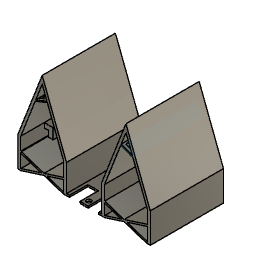
V shape load bearer v7 (Autodesk Fusion 360 design; units mm, degrees)
Autodesk Fusion 360 part; units mm, degrees
sketch "Sketch1" plane through (0, 0, 0) normal (0, 0, 1) x (1, 0, 0)
  line L0 (0, 0) -> (66, 0)
  line L1 (66, 0) -> (66, 150)
  line L2 (66, 150) -> (0, 150)
  line L3 (0, 150) -> (0, 0)
  dimension "d3" = 150
  dimension "d4" = 66
  constraint horizontal L0
  constraint vertical L1
  constraint horizontal L2
  constraint vertical L3
  constraint coincident L0.start L3.end
  measures "d3" distance of L0.start L2.end
  measures "d4" distance of L0.start L0.end
extrude "Extrude1" add sketch "Sketch1" along normal blind 2 makes body 1
sketch "Sketch2" plane through (0, 0, 2) normal (0, 0, 1) x (-1, 0, 0)
  line L0 (0, -150) -> (0, 0)
  line L1 (0, 0) -> (-66, 0)
  line L2 (-66, 0) -> (-66, -150)
  line L3 (-66, -150) -> (0, -150)
  line L4 (0, 0) -> (-3, 0)
  line L5 (-3, 0) -> (-3, -150)
  line L6 (-3, -150) -> (0, -150)
  line L7 (0, -150) -> (0, 0)
  line L8 (-66, -150) -> (-63, -150)
  line L9 (-63, -150) -> (-63, 0)
  line L10 (-63, 0) -> (-66, 0)
  line L11 (-66, 0) -> (-66, -150)
  dimension "d5" = 3
  dimension "d6" = 3
  constraint horizontal L4
  constraint vertical L5
  constraint horizontal L6
  constraint vertical L7
  constraint coincident L3 L5.end
  constraint coincident L0.end L1.start
  constraint horizontal L8
  constraint vertical L9
  constraint horizontal L10
  constraint vertical L11
  constraint coincident L1 L9.end
  constraint coincident L2.end L3.start
  measures "d5" distance of L0.end L4.end
  measures "d6" distance of L2.end L8.end
extrude "Extrude2" add sketch "Sketch2" along normal blind 40 contours L0 L1 L3 L4 L5 L6 L7 | L1 L2 L3 L8 L9 L10 L11 bodies 1
extrude "Extrude3" add 1 faces at (0, 100, 28) along direction (-1, 0, 0) blind 60 on bodies 1 bodies 1
extrude "Extrude4" add 1 faces at (66, 50, 28) along direction (1, 0, 0) blind 60 on bodies 1 bodies 1
sketch "Sketch3" plane through (0, 0, 0) normal (0, 0, -1) x (1, 0, 0)
  line L0 (-60, -150) -> (126, -150)
  line L1 (126, -150) -> (126, 0)
  line L2 (126, 0) -> (-60, 0)
  line L3 (-60, 0) -> (-60, -150)
  line L4 (-50, -10) -> (0, -10)
  line L5 (0, -10) -> (0, -140)
  line L6 (0, -140) -> (-50, -140)
  line L7 (-50, -140) -> (-50, -10)
  constraint horizontal L4
  constraint vertical L5
  constraint horizontal L6
  constraint vertical L7
extrude "Extrude5" cut sketch "Sketch3" against normal blind 38 contours L4 L5 L6 L7 bodies 1
extrude "Extrude6" cut 1 faces at (-50, 96.6667, 12.6667) along direction (-1, 0, 0) blind 5 on bodies 1 bodies 1
extrude "Extrude7" add 1 faces at (0, 53.3333, 12.6667) along direction (-1, 0, 0) blind 2 on bodies 1 bodies 1
extrude "Extrude8" add 1 faces at (-60, 100, 28) along direction (-1, 0, 0) blind 20 on bodies 1 bodies 1
extrude "Extrude9" cut 1 faces at (-55, 96.6667, 12.6667) along direction (-1, 0, 0) blind 20 on bodies 1 bodies 1
extrude "Extrude10" add 1 faces at (-75, 96.6667, 12.6667) along direction (1, 0, 0) blind 1 on bodies 1 bodies 1
extrude "Extrude11" cut 1 faces at (-26, 10, 12.6667) along direction (0, -1, 0) blind 5 on bodies 1 bodies 1
extrude "Extrude12" cut 1 faces at (-26, 140, 12.6667) along direction (0, 1, 0) blind 5 on bodies 1 bodies 1
sketch "Sketch4" plane through (0, 0, 0) normal (0, 0, -1) x (1, 0, 0)
  line L0 (-74, -145) -> (-74, -5)
  line L1 (-74, -5) -> (-2, -5)
  line L2 (-2, -5) -> (-2, -145)
  line L3 (-2, -145) -> (-74, -145)
  line L4 (-80, -150) -> (126, -150)
  line L5 (126, -150) -> (126, 0)
  line L6 (126, 0) -> (-80, 0)
  line L7 (-80, 0) -> (-80, -150)
extrude "Extrude13" cut 1 faces at (-74, 51.6667, 25.3333) along direction (-1, 0, 0) blind 1 on bodies 1 bodies 1
extrude "Extrude14" add 1 faces at (43, 50, 2) along direction (0, 0, -1) blind 5 on bodies 1 bodies 1
extrude "Extrude15" add 1 faces at (43, 50, 2) along direction (0, 0, 1) blind 3 on bodies 1 bodies 1
sketch "Sketch5" plane through (0, 0, 0) normal (0, 0, -1) x (1, 0, 0)
  line L0 (-75, -5) -> (-2, -5)
  line L1 (-2, -5) -> (-2, -145)
  line L2 (-2, -145) -> (-75, -145)
  line L3 (-75, -145) -> (-75, -5)
  line L4 (3, -150) -> (3, 0)
  line L5 (3, 0) -> (-80, 0)
  line L6 (-80, 0) -> (-80, -150)
  line L7 (-80, -150) -> (3, -150)
  line L8 (63, -150) -> (68, -150)
  line L9 (68, -150) -> (68, -145)
  line L10 (68, -145) -> (141, -145)
  line L11 (141, -145) -> (141, -5)
  line L12 (141, -5) -> (68, -5)
  line L13 (68, -5) -> (68, -145)
  dimension "d35" = 5
  dimension "d36" = 73
  dimension "d37" = 140
  constraint perpendicular L1 L8
  constraint perpendicular L8 L9
  constraint horizontal L10
  constraint vertical L11
  constraint horizontal L12
  constraint vertical L13
  measures "d35" distance of L8.end L9.end
  measures "d36" distance of L9.end L10.end
  measures "d37" distance of L9.end L12.end
extrude "Extrude16" add 1 faces at (126, 50, 28) along direction (1, 0, 0) blind 25 on bodies 1 bodies 1
extrude "Extrude17" cut 1 faces at (151, 50, 28) along direction (-1, 0, 0) blind 5 on bodies 1 bodies 1
extrude "Extrude18" cut sketch "Sketch5" against normal blind 38 contours L10 L11 L12 L13 bodies 1
sketch "Sketch6" plane through (0, 0, -3) normal (0, 0, -1) x (1, 0, 0)
  line L0 (63, -150) -> (63, 0)
  line L1 (63, 0) -> (3, 0)
  line L2 (3, 0) -> (3, -150)
  line L3 (3, -150) -> (63, -150)
  line L4 (33, 0) -> (33, -8)
  line L5 (33, -8) -> (33, -142)
  line L6 (33, -142) -> (33, -150)
  circle A0 centre (33, -142) radius 4
  circle A1 centre (33, -8) radius 4
  dimension "d44" = 8
  dimension "d45" = 134
  dimension "d46" = 8
  dimension "d47" = 8
  constraint midpoint L1 L4.start
  constraint perpendicular L1 L4
  constraint perpendicular L1 L5
  constraint midpoint L3 L6.end
  constraint coincident L5.end L6.start
  constraint coincident L4.end L5.start
  measures "d44" distance of L4.start L4.end
  measures "d45" distance of L4.end L5.end
  measures "d46" diameter of A0
  measures "d47" diameter of A1
extrude "Extrude19" cut sketch "Sketch6" against normal blind 10 contours L5 L6 A0 | L5 L6 A0 | L4 L5 A1 | L4 L5 A1 bodies 1
sketch "Sketch7" plane through (0, 0, -3) normal (0, 0, -1) x (1, 0, 0)
  circle A0 centre (33, -142) radius 4
  circle A1 centre (33, -8) radius 4
  line L0 (63, -150) -> (63, 0)
  line L1 (63, 0) -> (3, 0)
  line L2 (3, 0) -> (3, -150)
  line L3 (3, -150) -> (63, -150)
  line L4 (63, -132.342) -> (58, -132.342)
  line L5 (33, -142) -> (33, -132)
  line L6 (33, -8) -> (33, -18)
  line L7 (58, -132) -> (8, -132)
  line L8 (8, -132) -> (8, -18)
  line L9 (8, -18) -> (58, -18)
  line L10 (58, -18) -> (58, -132)
  line L11 (33, -8) -> (33, 0)
  dimension "d50" = 5
  dimension "d51" = 10
  dimension "d52" = 10
  dimension "d53" = 50
  dimension "d54" = 114
  constraint coincident L0 L4.start
  constraint perpendicular L0 L4
  constraint coincident A0.centre L5.start
  constraint vertical L5
  constraint coincident A1.centre L6.start
  constraint vertical L6
  constraint horizontal L7
  constraint vertical L8
  constraint horizontal L9
  constraint vertical L10
  constraint midpoint L1 L11.end
  measures "d50" distance of L4.start L4.end
  measures "d51" distance of A0.centre L5.end
  measures "d52" distance of A1.centre L6.end
  measures "d53" distance of L7.start L7.end
  measures "d54" distance of L7.start L9.end
extrude "Extrude20" cut sketch "Sketch7" against normal blind 10 contours L7 L8 L9 L10 bodies 1
sketch "Sketch8" plane through (0, 150, 0) normal (0, 1, 0) x (-1, 0, 0)
  line L0 (-146, 42) -> (-146, 0)
  line L1 (-146, 0) -> (-63, 0)
  line L2 (-63, 0) -> (-63, -3)
  line L3 (-63, -3) -> (-3, -3)
  line L4 (-3, -3) -> (-3, 0)
  line L5 (-3, 0) -> (80, 0)
  line L6 (80, 0) -> (80, 42)
  line L7 (80, 42) -> (-3, 42)
  line L8 (-3, 42) -> (-3, 5)
  line L9 (-3, 5) -> (-63, 5)
  line L10 (-63, 5) -> (-63, 42)
  line L11 (-63, 42) -> (-146, 42)
  line L12 (80, 0) -> (-3, 0)
  line L13 (-3, 0) -> (-3, 42)
  line L14 (-3, 42) -> (80, 42)
  line L15 (80, 42) -> (80, 0)
  line L16 (-63, 42) -> (-146, 42)
  line L17 (-146, 42) -> (-146, 0)
  line L18 (-146, 0) -> (-63, 0)
  line L19 (-63, 0) -> (-63, 42)
  constraint horizontal L12
  constraint vertical L13
  constraint horizontal L14
  constraint vertical L15
  constraint coincident L7.end L8.start
  constraint coincident L5.end L6.start
  constraint horizontal L16
  constraint vertical L17
  constraint horizontal L18
  constraint vertical L19
  constraint coincident L0.end L1.start
  constraint coincident L10.end L11.start
extrude "Extrude21" add 1 faces at (-50.6667, 145, 25.3333) along direction (0, -1, 0) blind 25 on bodies 1 bodies 1
extrude "Extrude22" add 1 faces at (92.3333, 145, 25.3333) along direction (0, -1, 0) blind 25 on bodies 1 bodies 1
extrude "Extrude23" cut sketch "Sketch8" against normal blind 25 contours L0 L1 L10 L11 L16 L17 L18 L19 | L5 L6 L7 L8 L12 L13 L14 L15 bodies 1
extrude "Extrude24" cut 1 faces at (116.6667, 5, 25.3333) along direction (0, -1, 0) blind 10 on bodies 1 bodies 1
extrude "Extrude25" cut 1 faces at (92.3333, 120, 25.3333) along direction (0, 1, 0) blind 10 on bodies 1 bodies 1
extrude "Extrude26" cut 1 faces at (-50.6667, 120, 25.3333) along direction (0, 1, 0) blind 10 on bodies 1 bodies 1
extrude "Extrude27" cut 1 faces at (-26.3333, 5, 12.6667) along direction (0, -1, 0) blind 10 on bodies 1 bodies 1
extrude "Extrude28" cut 2 faces at (92.3333, 83.3333, 38) (-50.6667, 83.3333, 38) along direction (0, 0, 1) blind 10 on bodies 1 bodies 1 makes body 2 at (141, 83.3333, 14) makes body 3 at (-75, 83.3333, 14)
sketch "Sketch9" plane through (0, 125, 0) normal (0, 1, 0) x (-1, 0, 0)
  line L0 (2, 0) -> (2, 42)
  line L1 (2, 42) -> (-3, 42)
  line L2 (-3, 42) -> (-3, 5)
  line L3 (-3, 5) -> (-3, 0)
  line L4 (-3, 0) -> (2, 0)
  line L5 (2, 42) -> (2, 40)
  line L6 (2, 40) -> (75, 0)
  line L7 (75, 0) -> (75, 2)
  line L8 (75, 2) -> (2, 42)
  line L9 (2, 0) -> (2, 2)
  line L10 (2, 2) -> (75, 41.9933)
  line L11 (75, 41.9933) -> (75, 39.9933)
  line L12 (75, 39.9933) -> (2, 0)
  dimension "d73" = 2
  dimension "d74" = 2
  dimension "d75" = 2
  constraint coincident L0.end L1.start
  constraint coincident L0 L5.end
  constraint perpendicular L1 L5
  constraint parallel L0 L7
  constraint parallel L6 L8
  constraint coincident L0.start L4.end
  constraint coincident L0 L9.end
  constraint parallel L9 L11
  measures "d73" distance of L6.end L7.end
  measures "d74" distance of L0.start L9.end
  measures "d75" distance of L10.end L11.end
extrude "Extrude43" cut 1 faces at (52.6518, 8.4679, -3) along direction (0, 0, 1) blind 7 on bodies 1 bodies 1
extrude "Extrude44" add 1 faces at (52.6518, 8.4679, 4) along direction (0, 0, -1) blind 2 on bodies 1 bodies 1
extrude "Extrude45" cut 2 faces at (-0.3333, 41.6667, 0) (64.6667, 83.3333, 0) along direction (0, 0, 1) blind 2 on bodies 1 bodies 1
sketch "Sketch19" plane through (-75, 0, 0) normal (1, 0, 0) x (0, 1, 0)
  line L0 (0, 42) -> (0, 0)
  line L1 (0, 0) -> (125, 0)
  line L2 (125, 0) -> (125, 42)
  line L3 (125, 42) -> (0, 42)
  line L4 (85, 51) -> (40, 51)
  line L5 (40, 51) -> (40, 33)
  line L6 (40, 33) -> (85, 33)
  line L7 (85, 33) -> (85, 51)
  line L8 (85, 51) -> (40, 33) construction
  line L9 (40, 51) -> (85, 33) construction
  point P0 (62.5, 42)
  dimension "d122" = 45
  dimension "d127" = 18
  constraint horizontal L4
  constraint perpendicular L4 L5
  constraint parallel L4 L6
  constraint parallel L5 L7
  constraint coincident L8 P0
  constraint coincident L9 P0
  constraint midpoint L3 P0
  measures "d122" distance of L5.end L6.end
  measures "d127" distance of L4.end L5.end
extrude "Extrude46" add sketch "Sketch19" along normal blind 15 contours L3 L4 L5 L7 | L3 L5 L6 L7 bodies 3
sketch "Sketch20" plane through (141, 0, 0) normal (-1, 0, 0) x (0, -1, 0)
  line L0 (-125, 0) -> (0, 0)
  line L1 (0, 0) -> (0, 42)
  line L2 (0, 42) -> (-125, 42)
  line L3 (-125, 42) -> (-125, 0)
  line L4 (-40, 51) -> (-85, 51)
  line L5 (-85, 51) -> (-85, 33)
  line L6 (-85, 33) -> (-40, 33)
  line L7 (-40, 33) -> (-40, 51)
  line L8 (-40, 51) -> (-85, 33) construction
  line L9 (-85, 51) -> (-40, 33) construction
  point P0 (-62.5, 42)
  dimension "d125" = 45
  dimension "d126" = 18
  constraint horizontal L4
  constraint perpendicular L4 L5
  constraint parallel L4 L6
  constraint parallel L5 L7
  constraint coincident L8 P0
  constraint coincident L9 P0
  constraint midpoint L2 P0
  measures "d125" distance of L5.end L6.end
  measures "d126" distance of L4.start L6.end
extrude "Extrude47" add sketch "Sketch20" along normal blind 15 contours L2 L4 L5 L7 | L2 L5 L6 L7 bodies 2
extrude "Extrude48" add 4 faces at (144.3333, 55, 42) (64.6667, 41.6667, 42) (1.3333, 83.3333, 42) (-78.3333, 55, 42) along direction (0, 0, 1) blind 9 on bodies 1 2 3 bodies 2 1 3
sketch "Sketch21" plane through (0, 0, 0) normal (0, -1, 0) x (1, 0, 0)
  line L0 (-2, 2) -> (68, 2)
  line L1 (68, 2) -> (68, 51)
  line L2 (68, 51) -> (63, 51)
  line L3 (63, 51) -> (63, 5)
  line L4 (63, 5) -> (3, 5)
  line L5 (3, 5) -> (3, 51)
  line L6 (3, 51) -> (-2, 51)
  line L7 (-2, 51) -> (-2, 2)
  line L8 (68, 51) -> (141, 51)
  line L9 (141, 51) -> (104.5, 51)
  line L10 (104.5, 51) -> (104.5, 151)
  line L11 (104.5, 151) -> (104.5, 146)
  line L12 (68, 51) -> (104.5, 146)
  line L13 (63, 51) -> (104.5, 159.0137)
  line L14 (104.5, 159.0137) -> (104.5, 151)
  line L15 (104.5, 159.0137) -> (145.9959, 51)
  line L16 (145.9959, 51) -> (140.9959, 51)
  line L17 (140.9959, 51) -> (104.5, 146)
  dimension "d132" = 100
  dimension "d133" = 5
  dimension "d134" = 5
  constraint coincident L1.end L2.start
  constraint perpendicular L1 L8
  constraint midpoint L8 L9.end
  constraint perpendicular L9 L10
  constraint parallel L10 L11
  constraint coincident L2.end L3.start
  constraint parallel L12 L13
  constraint parallel L11 L14
  constraint perpendicular L14 L16
  measures "d132" distance of L9.end L10.end
  measures "d133" distance of L10.end L11.end
  measures "d134" distance of L15.end L16.end
extrude "Extrude49" add sketch "Sketch21" against normal blind 125 contours L2 L10 L11 L12 L13 L14 | L8 L9 L10 L11 L14 L15 L16 L17 bodies 1 2
sketch "Sketch22" plane through (0, 0, 33) normal (0, 0, -1) x (1, 0, 0)
  line L0 (141, -85) -> (141, -40)
  line L1 (141, -40) -> (126, -40)
  line L2 (126, -40) -> (126, -85)
  line L3 (126, -85) -> (141, -85)
  line L4 (141, -40) -> (133.5, -40)
  line L5 (133.5, -40) -> (133.5, -85)
  line L6 (133.5, -85) -> (141, -85)
  line L7 (141, -85) -> (141, -40)
  line L8 (-75, -40) -> (-67.5, -40)
  line L9 (-67.5, -40) -> (-67.5, -85)
  line L10 (-67.5, -85) -> (-75, -85)
  line L11 (-75, -85) -> (-75, -40)
  dimension "d137" = 7.5
  constraint horizontal L4
  constraint vertical L5
  constraint horizontal L6
  constraint vertical L7
  constraint midpoint L3 L5.end
  constraint coincident L0.end L1.start
  constraint horizontal L8
  constraint vertical L9
  constraint horizontal L10
  constraint vertical L11
  measures "d137" distance of L8.start L8.end
extrude "Extrude50" cut sketch "Sketch22" against normal blind 10 contours L0 L1 L3 L4 L5 L6 L7 | L8 L9 L10 L11 bodies 1 3
sketch "Sketch23" plane through (0, 150, 0) normal (0, 1, 0) x (-1, 0, 0)
  line L0 (-3, 2) -> (-3, 5)
  line L1 (-3, 5) -> (-63, 5)
  line L2 (-63, 5) -> (-63, 2)
  line L3 (-63, 2) -> (-3, 2)
  line L4 (-3, 5) -> (-33, 5)
  line L5 (-33, 5) -> (-33, -15)
  line L6 (-33, -15) -> (-33, 92.0217)
  line L7 (-33, 92.0217) -> (100, 92.0217)
  line L8 (100, 92.0217) -> (100, -15)
  line L9 (100, -15) -> (-33, -15)
  constraint coincident L0.end L1.start
  constraint midpoint L1 L4.end
  constraint perpendicular L4 L5
  constraint perpendicular L1 L6
  constraint perpendicular L6 L7
  constraint perpendicular L1 L8
  constraint perpendicular L5 L9
extrude "Extrude51" cut sketch "Sketch23" against normal blind 150 contours L0 L1 L3 L4 L5 L6 L7 L8 L9 bodies 1 3
extrude "Extrude52" cut 1 faces at (3, 100, 3) along direction (1, 0, 0) blind 30 on bodies 1 bodies 1
sketch "Sketch24" plane through (0, 125, 0) normal (0, 1, 0) x (-1, 0, 0)
  line L0 (-68, 2) -> (-63, 2)
  line L1 (-63, 2) -> (-63, 5)
  line L2 (-63, 5) -> (-63, 51)
  line L3 (-63, 51) -> (-104.5, 159.0137)
  line L4 (-104.5, 159.0137) -> (-145.9959, 51)
  line L5 (-145.9959, 51) -> (-146, 51)
  line L6 (-146, 51) -> (-146, 0)
  line L7 (-146, 0) -> (-141, 0)
  line L8 (-141, 0) -> (-141, 51)
  line L9 (-141, 51) -> (-140.9959, 51)
  line L10 (-140.9959, 51) -> (-104.5, 146)
  line L11 (-104.5, 146) -> (-68, 51)
  line L12 (-68, 51) -> (-68, 2)
  line L13 (-68, 2) -> (-68, 5)
  line L14 (-68, 2) -> (-141, 25.5)
  line L15 (-141, 25.5) -> (-140.0807, 28.3557)
  line L16 (-140.0807, 28.3557) -> (-68, 5)
  line L17 (-141, 0) -> (-141, 3)
  line L18 (-141, 3) -> (-68, 26.5)
  line L19 (-68, 26.5) -> (-67.0807, 23.6443)
  line L20 (-67.0807, 23.6443) -> (-141, 0)
  line L21 (-140.0807, 28.3557) -> (-141.8096, 28.9122)
  line L22 (-141.8096, 28.9122) -> (-142.7286, 26.0575)
  line L23 (-142.7286, 26.0575) -> (-141, 25.5)
  dimension "d144" = 3
  dimension "d145" = 3
  dimension "d146" = 3
  constraint coincident L0.start L12.end
  constraint coincident L12 L13.end
  constraint perpendicular L0 L13
  constraint midpoint L8 L14.end
  constraint perpendicular L14 L15
  constraint coincident L7.end L8.start
  constraint coincident L8 L17.end
  constraint midpoint L12 L18.end
  constraint perpendicular L18 L19
  constraint perpendicular L15 L21
  constraint perpendicular L21 L22
  measures "d144" distance of L14.end L15.end
  measures "d145" distance of L7.end L17.end
  measures "d146" distance of L18.end L19.end
extrude "Extrude53" add sketch "Sketch24" against normal blind 125 contours L12 L13 L14 L16 L20 | L8 L14 L17 L18 L20 | L14 L16 L18 L20 | L12 L16 L18 L20 | L14 L15 L16 L18 | L8 L15 L21 bodies 1 3
sketch "Sketch25" plane through (0, 125, 0) normal (0, 1, 0) x (-1, 0, 0)
  line L0 (-141, 28.6516) -> (-141, 51)
  line L1 (-141, 51) -> (-140.9959, 51)
  line L2 (-140.9959, 51) -> (-104.5, 146)
  line L3 (-104.5, 146) -> (-68, 51)
  line L4 (-68, 51) -> (-68, 26.5)
  line L5 (-68, 26.5) -> (-101.2849, 15.785)
  line L6 (-101.2849, 15.785) -> (-140.0807, 28.3557)
  line L7 (-140.0807, 28.3557) -> (-141, 28.6516)
  line L8 (-141, 25.5) -> (-106.0532, 14.25)
  line L9 (-106.0532, 14.25) -> (-141, 3)
  line L10 (-141, 3) -> (-141, 25.5)
  line L11 (-141, 0) -> (-101.267, 12.7093)
  line L12 (-101.267, 12.7093) -> (-68, 2)
  line L13 (-68, 2) -> (-63, 2)
  line L14 (-63, 2) -> (-63, 5)
  line L15 (-63, 5) -> (-63, 51)
  line L16 (-63, 51) -> (-104.5, 159.0137)
  line L17 (-104.5, 159.0137) -> (-145.9959, 51)
  line L18 (-145.9959, 51) -> (-146, 51)
  line L19 (-146, 51) -> (-146, 0)
  line L20 (-146, 0) -> (-141, 0)
  line L21 (-68, 5) -> (-96.4992, 14.2343)
  line L22 (-96.4992, 14.2343) -> (-68, 23.3503)
  line L23 (-68, 23.3503) -> (-68, 5)
  line L24 (-96.3743, 124.8508) -> (-95.657, 122.9839)
  line L25 (-95.657, 122.9839) -> (-116.9083, 114.8189)
  line L26 (-96.3743, 124.8508) -> (-117.4972, 116.7352)
  line L27 (-117.4972, 116.7352) -> (-116.9083, 114.8189)
  dimension "d149" = 2
  constraint coincident L3 L24.start
  constraint perpendicular L24 L25
  constraint perpendicular L24 L26
  measures "d149" distance of L24.start L24.end
extrude "Extrude54" add sketch "Sketch25" against normal blind 125 contours L2 L3 L24 L25 L26 bodies 1
sketch "Sketch26" plane through (53.4781, 0, 139.1895) normal (-0.35865, 0, -0.933472) x (0, -1, 0)
  line L0 (-125, -45.185) -> (-125, -67.411)
  line L1 (-125, -67.411) -> (0, -67.411)
  line L2 (0, -67.411) -> (0, -45.185)
  line L3 (0, -45.185) -> (-125, -45.185)
  line L4 (-5, -62) -> (-10, -62)
  line L5 (-10, -62) -> (-10, -50)
  line L6 (-10, -50) -> (-5, -50)
  line L7 (-5, -50) -> (-5, -62)
  constraint horizontal L4
  constraint vertical L5
  constraint horizontal L6
  constraint vertical L7
extrude "Extrude55" cut sketch "Sketch26" against normal blind 5 contours L4 L5 L6 L7 bodies 1
sketch "Sketch27" plane through (53.4781, 0, 139.1895) normal (-0.35865, 0, -0.933472) x (0, -1, 0)
  line L0 (-10, -62) -> (-10, -50)
  line L1 (-10, -50) -> (-5, -50)
  line L2 (-5, -50) -> (-5, -62)
  line L3 (-5, -62) -> (-10, -62)
  line L4 (-125, -45.185) -> (-125, -67.411)
  line L5 (-125, -67.411) -> (0, -67.411)
  line L6 (0, -67.411) -> (0, -45.185)
  line L7 (0, -45.185) -> (-125, -45.185)
extrude "Extrude56" cut 1 faces at (107.8586, 10, 119.0101) along direction (0, 1, 0) blind 110 on bodies 1 bodies 1
extrude "Extrude57" cut 1 faces at (100.3908, 81.6667, 121.8793) along direction (-0.933472, 0, 0.35865) blind 2 on bodies 1 bodies 1
extrude "Extrude58" cut 1 faces at (111.5924, 43.3333, 117.5755) along direction (0.933472, 0, -0.35865) blind 2 on bodies 1 bodies 1
sketch "Sketch28" plane through (53.4781, 0, 139.1895) normal (-0.35865, 0, -0.933472) x (0, -1, 0)
  line L0 (-125, -45.185) -> (-125, -67.411)
  line L1 (-125, -67.411) -> (0, -67.411)
  line L2 (0, -67.411) -> (0, -45.185)
  line L3 (0, -45.185) -> (-125, -45.185)
  line L4 (-5, -48) -> (-5, -64)
  line L5 (-5, -64) -> (-120, -64)
  line L6 (-120, -64) -> (-120, -48)
  line L7 (-120, -48) -> (-5, -48)
ref_plane "WorkPlane1" through (33, 148, 3.5) normal (-1, 0, 0) x (0, 0, 1)
mirror "Mirror1" about plane through (33, 148, 3.5) normal (-1, 0, 0) of bodies 1 merged
sketch "Sketch29" plane through (0, 0, 2) normal (0, 0, -1) x (1, 0, 0)
  circle A0 centre (33, -8) radius 4
  line L0 (8, -18) -> (58, -18)
  line L1 (58, -18) -> (58, -132)
  line L2 (58, -132) -> (8, -132)
  line L3 (8, -132) -> (8, -18)
  line L4 (68, 0) -> (-2, 0)
  line L5 (-2, 0) -> (-2, -125)
  line L6 (-2, -125) -> (3, -125)
  line L7 (3, -125) -> (3, -150)
  line L8 (3, -150) -> (63, -150)
  line L9 (63, -150) -> (63, -125)
  line L10 (63, -125) -> (68, -125)
  line L11 (68, -125) -> (68, 0)
  circle A1 centre (33, -142) radius 4
  line L12 (8, -18) -> (26, -18)
  line L13 (26, -18) -> (26, -5)
  line L14 (26, -5) -> (8, -5)
  line L15 (8, -5) -> (8, -18)
  line L16 (58, -18) -> (40, -18)
  line L17 (40, -18) -> (40, -5)
  line L18 (40, -5) -> (58, -5)
  line L19 (58, -5) -> (58, -18)
  line L20 (8, -132) -> (26, -132)
  line L21 (26, -132) -> (26, -145)
  line L22 (26, -145) -> (8, -145)
  line L23 (8, -145) -> (8, -132)
  line L24 (58, -132) -> (40, -132)
  line L25 (40, -132) -> (40, -145)
  line L26 (40, -145) -> (58, -145)
  line L27 (58, -145) -> (58, -132)
  dimension "d163" = 18
  dimension "d164" = 18
  dimension "d165" = 18
  dimension "d166" = 13
  dimension "d167" = 18
  constraint horizontal L12
  constraint vertical L13
  constraint horizontal L14
  constraint vertical L15
  constraint coincident L0.start L3.end
  constraint horizontal L16
  constraint vertical L17
  constraint horizontal L18
  constraint vertical L19
  constraint coincident L0.end L1.start
  constraint horizontal L20
  constraint vertical L21
  constraint horizontal L22
  constraint vertical L23
  constraint coincident L2.end L3.start
  constraint horizontal L24
  constraint vertical L25
  constraint horizontal L26
  constraint vertical L27
  constraint coincident L1.end L2.start
  measures "d163" distance of L0.start L12.end
  measures "d164" distance of L0.end L16.end
  measures "d165" distance of L2.end L20.end
  measures "d166" distance of L2.end L22.end
  measures "d167" distance of L1.end L24.end
extrude "Extrude59" cut sketch "Sketch29" against normal blind 10 contours L0 L12 L13 L14 L15 | L2 L20 L21 L22 L23 | L0 L16 L17 L18 L19 | L2 L24 L25 L26 L27 bodies 1
extrude "Extrude60" cut 2 faces at (28.3333, 18, 3) (37.6667, 18, 3) along direction (0, -1, 0) blind 3 on bodies 1 bodies 1
extrude "Extrude61" cut 2 faces at (35.3333, 132, 3) (28.3333, 132, 3) along direction (0, 1, 0) blind 3 on bodies 1 bodies 1
extrude "Extrude62" add 1 faces at (30.6667, 135, 3) along direction (0, -1, 0) blind 120 on bodies 1 bodies 1
extrude "Extrude63" cut 1 faces at (20, 145, 3) along direction (0, 1, 0) blind 7 on bodies 1 bodies 1
extrude "Extrude64" cut 1 faces at (46, 145, 3) along direction (0, 1, 0) blind 18 on bodies 1 bodies 1
extrude "Extrude65" cut 2 faces at (46, 5, 3) (20, 5, 3) along direction (0, -1, 0) blind 16 on bodies 1 bodies 1 makes body 4 at (-10.8333, 41.6667, 87.0046) makes body 5 at (76.8333, 41.6667, 87.0046)
sketch "Sketch30" plane through (0, 0, 2) normal (0, 0, -1) x (1, 0, 0)
  line L0 (40, -150) -> (40, 0)
  line L1 (40, 0) -> (26, 0)
  line L2 (26, 0) -> (26, -150)
  line L3 (26, -150) -> (40, -150)
  circle A0 centre (33, -8) radius 4
  circle A1 centre (33, -142) radius 4
  line L4 (33, -142) -> (33, -118.5)
  line L5 (33, -118.5) -> (8, -118.5)
  line L6 (8, -118.5) -> (8, -113)
  line L7 (8, -113) -> (60, -113)
  line L8 (60, -113) -> (60, -118.5)
  line L9 (60, -118.5) -> (33, -118.5)
  line L10 (33, -8) -> (33, -31.5)
  line L11 (33, -31.5) -> (6.7662, -31.5)
  line L12 (6.7662, -31.5) -> (6.7662, -37)
  line L13 (6.7662, -37) -> (61.566, -37)
  line L14 (33, -31.5) -> (60.9929, -31.5)
  line L15 (60.9929, -31.5) -> (60.9929, -38.1223)
  dimension "d182" = 23.5
  dimension "d183" = 23.5
  dimension "d184" = 5.5
  constraint coincident A1.centre L4.start
  constraint parallel L0 L4
  constraint perpendicular L2 L5
  constraint perpendicular L5 L6
  constraint perpendicular L6 L7
  constraint perpendicular L7 L8
  constraint perpendicular L4 L9
  constraint coincident A0.centre L10.start
  constraint parallel L2 L10
  constraint perpendicular L2 L11
  constraint perpendicular L11 L12
  constraint perpendicular L12 L13
  constraint perpendicular L10 L14
  constraint perpendicular L11 L15
  measures "d182" distance of A1.centre L4.end
  measures "d183" distance of A0.centre L10.end
  measures "d184" distance of L11.end L12.end
extrude "Extrude66" add sketch "Sketch30" against normal blind 3 contours L0 L7 L8 L9 | L2 L5 L6 L7 | L0 L13 L14 L15 | L2 L11 L12 L13 bodies 4 1 5
sketch "Sketch31" plane through (0, 0, 2) normal (0, 0, -1) x (1, 0, 0)
  line L0 (40, -31.5) -> (40, 0)
  line L1 (40, 0) -> (26, 0)
  line L2 (26, 0) -> (26, -31.5)
  line L3 (26, -31.5) -> (8, -31.5)
  line L4 (8, -31.5) -> (8, 0)
  line L5 (8, 0) -> (-2, 0)
  line L6 (-2, 0) -> (-2, -125)
  line L7 (-2, -125) -> (3, -125)
  line L8 (3, -125) -> (3, -150)
  line L9 (3, -150) -> (8, -150)
  line L10 (8, -150) -> (8, -118.5)
  line L11 (8, -118.5) -> (26, -118.5)
  line L12 (26, -118.5) -> (26, -150)
  line L13 (26, -150) -> (40, -150)
  line L14 (40, -150) -> (40, -118.5)
  line L15 (40, -118.5) -> (58, -118.5)
  line L16 (58, -118.5) -> (58, -150)
  line L17 (58, -150) -> (63, -150)
  line L18 (63, -150) -> (63, -125)
  line L19 (63, -125) -> (68, -125)
  line L20 (68, -125) -> (68, 0)
  line L21 (68, 0) -> (58, 0)
  line L22 (58, 0) -> (58, -31.5)
  line L23 (58, -31.5) -> (40, -31.5)
  circle A0 centre (33, -142) radius 4
  circle A1 centre (33, -8) radius 4
  line L24 (40, -37) -> (58, -37)
  line L25 (58, -37) -> (58, -113)
  line L26 (58, -113) -> (40, -113)
  line L27 (40, -113) -> (40, -37)
  line L28 (26, -37) -> (26, -113)
  line L29 (26, -113) -> (8, -113)
  line L30 (8, -113) -> (8, -37)
  line L31 (8, -37) -> (26, -37)
  line L32 (58, -78.1246) -> (-6, -78.1246)
  line L33 (-6, -78.1246) -> (-6, -71.8754)
  line L34 (-6, -71.8754) -> (58, -71.8754)
  line L35 (58, -71.8754) -> (58, -78.1246)
  line L36 (58, -78.1246) -> (-6, -71.8754) construction
  line L37 (-6, -78.1246) -> (58, -71.8754) construction
  point P0 (26, -75)
  constraint horizontal L32
  constraint perpendicular L32 L33
  constraint parallel L32 L34
  constraint parallel L33 L35
  constraint coincident L36 P0
  constraint coincident L37 P0
  constraint coincident L25 L32.start
  constraint midpoint L28 P0
extrude "Extrude67" add sketch "Sketch31" against normal blind 3 contours L28 L30 L32 L34 | L25 L27 L32 L34 L35 bodies 4
extrude "Extrude68" add 2 faces at (20, 78.1246, 4) (52, 78.1246, 3) along direction (0, 1, 0) blind 10 on bodies 4 bodies 4
extrude "Extrude69" add 2 faces at (14, 71.8754, 3) (46, 71.8754, 3) along direction (0, -1, 0) blind 10 on bodies 4 bodies 4
extrude "Extrude70" add 2 faces at (14, 113, 3) (46, 113, 3) along direction (0, -1, 0) blind 79 on bodies 4 bodies 4
